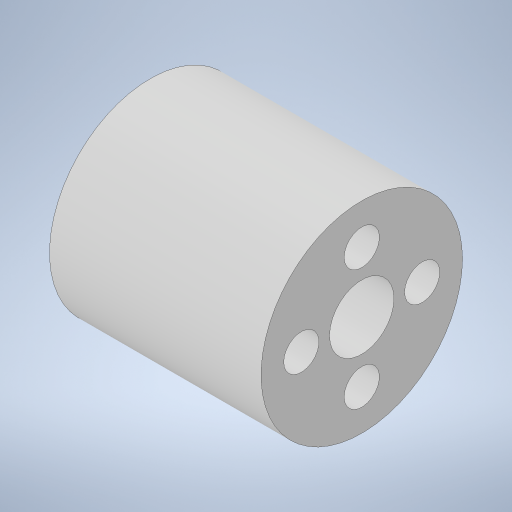
# Autodesk Inventor part: shoulder1_upper_enocder_spacer
Saved by Autodesk Inventor 2024 (Build 280153000, 153)
## iProperties
Created: 2025-08-06
Part Number: shoulder1_upper_enocder_spacer
Material: 一般
Document SubType Name: Modeling
Designer: HosodaLab2
Density: 1 g/cm^3
Appearance: 既定
Author: HosodaLab2
Autodesk Inventor part; units mm, degrees
ref_plane "YZ Plane" through (0, 0, 0) normal (1, 0, 0) x (0, 1, 0)
ref_plane "XZ Plane" through (0, 0, 0) normal (0, 1, 0) x (-1, 0, 0)
ref_plane "XY Plane" through (0, 0, 0) normal (0, 0, 1) x (1, 0, 0)
sketch "スケッチ1" plane through (0, 0, 0) normal (0, 1, 0) x (-1, 0, 0)
  circle A0 centre (0, 0) radius 3.2
  circle A1 centre (0, 0) radius 10
  dimension "d0" = 6.4
  dimension "d1" = 20
  constraints: 2 centre point, 2 coincident
  measures "d0" diameter of A0
  measures "d1" diameter of A1
extrude "押し出し1" add sketch "スケッチ1" along normal blind 21
sketch "スケッチ2" plane through (0, 21, 0) normal (0, 1, 0) x (1, 0, 0)
  circle A0 centre (0, 0) radius 6 construction
  point P0 (-6, 0)
  point P1 (0, -6)
  point P2 (6, 0)
  point P3 (0, 6)
  dimension "d4" = 12
  dimension "d7" = 360
  constraints: 1 coincident, 1 horizontal alignment, 7 other
hole "穴1" at (-6, 21, 0) at (0, 21, 6) at (6, 21, 0) at (0, 21, -6) direction (0, -1, 0) diameter 3.5 end through all
